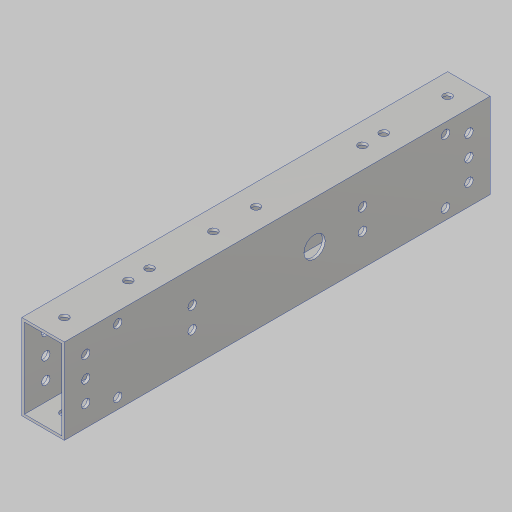
# Autodesk Inventor part: EL2-C-005
Saved by Autodesk Inventor 2023.5 (Build 275446000, 446)
## iProperties
RuleStatus: InUse
Created: 2025-01-11
Part Number: EL2-C-005
Material: Aluminum 6061
Document SubType Name: Modeling
Designer: brand
Mass: 304.185 g
Surface Area: 718.547 cm^2
Volume: 112.661 cm^3
Density: 2.7 g/cm^3
Appearance: Aluminum - Flat
AfterDocNew0: SHOW
AfterDocOpen0: SHOW
Author: brand
Autodesk Inventor part; units mm, degrees
ref_plane "YZ Plane" through (0, 0, 0) normal (1, 0, 0) x (0, 1, 0)
ref_plane "XZ Plane" through (0, 0, 0) normal (0, 1, 0) x (-1, 0, 0)
ref_plane "XY Plane" through (0, 0, 0) normal (0, 0, 1) x (1, 0, 0)
sketch "Sketch1" plane through (0, 0, 0) normal (0, 0, 1) x (1, 0, 0)
  line L0 (-12.7, -25.4) -> (12.7, -25.4)
  line L1 (12.7, -25.4) -> (12.7, 25.4)
  line L2 (12.7, 25.4) -> (-12.7, 25.4)
  line L3 (-12.7, 25.4) -> (-12.7, -25.4)
  line L4 (-12.7, -25.4) -> (12.7, 25.4) construction
  line L5 (12.7, -25.4) -> (-12.7, 25.4) construction
  line L6 (-11.1125, 23.8125) -> (11.1125, 23.8125)
  line L7 (11.1125, 23.8125) -> (11.1125, -23.8125)
  line L8 (11.1125, -23.8125) -> (-11.1125, -23.8125)
  line L9 (-11.1125, -23.8125) -> (-11.1125, 23.8125)
  point P0 (0, 0)
  dimension "width" = 25.4
  dimension "height" = 50.8
  dimension "thickness" = 1.5875
  constraints: 20 end point, 4 parallel, 2 midpoint, 2 perpendicular, 1 horizontal, 3 other
  measures "width" distance of L2.end L1.end
  measures "height" distance of L1.end L0.end
  measures "thickness" distance between parallel lines of L2 L6
extrude "Extrusion1" add sketch "Sketch1" along normal mid plane 254
sketch "Sketch2" plane through (-12.7, -25.4, 127) normal (-1, 0, 0) x (0, 0, 1)
  line L0 (-254, 0) -> (-254, 50.8) construction
  line L1 (-254, 50.8) -> (0, 50.8) construction
  line L2 (0, 50.8) -> (0, 0) construction
  line L3 (0, 0) -> (-254, 0) construction
  point P0 (-127, 25.4)
  point P1 (-241.3, 38.1)
  point P2 (-241.3, 25.4)
  point P3 (-241.3, 12.7)
  point P4 (-12.7, 38.1)
  point P5 (-12.7, 25.4)
  point P6 (-12.7, 12.7)
  point P7 (-254, 25.4)
  dimension "d5" = 12.7
  dimension "d6" = 12.7
  dimension "d7" = 12.7
  dimension "d8" = 12.7
  constraints: 4 horizontal alignment, 4 vertical alignment, 1 midpoint
  measures "d5" distance of point (-241.3, 38.1) point (-241.3, 25.4)
  measures "d6" distance of point (-241.3, 12.7) point (-241.3, 25.4)
  measures "d7" distance from line of L0 point (-241.3, 25.4)
  measures "d8" distance from line of L2 point (-12.7, 25.4)
hole "Block Mount Holes" at (-12.7, 12.7, -114.3) at (-12.7, 0, -114.3) at (-12.7, -12.7, -114.3) at (-12.7, 12.7, 114.3) at (-12.7, 0, 114.3) at (-12.7, -12.7, 114.3) direction (1, 0, 0) diameter 5.1054 end through all clearance for "Flat Head Machine Screw (82)" size "#10" standard "Ansi Unified Screw Threads"
sketch "Sketch4" plane through (-12.7, 25.4, 127) normal (0, 1, 0) x (1, 0, 0)
  line L0 (0, 254) -> (25.4, 254) projected
  line L1 (12.7, 190.5) -> (12.7, 63.5) construction
  point P0 (12.7, 127)
  point P1 (12.7, 254)
  point P2 (12.7, 203.2)
  point P3 (12.7, 50.8)
  point P4 (12.7, 127)
  dimension "d61" = 12.7
  dimension "d65" = 127
  dimension "d66" = 12.7
  constraints: 3 vertical alignment, 2 end point, 2 midpoint, 1 coincident, 1 vertical
  measures "d61" distance of point (12.7, 203.2) L1.start
  measures "d65" distance of L1.end L1.start
  measures "d66" distance of L1.end point (12.7, 50.8)
hole "Hole3" at (0, 25.4, 63.5) at (0, 25.4, -63.5) at (0, 25.4, -76.2) at (0, 25.4, 76.2) direction (0, -1, 0) diameter 5.1054 end through all clearance for "Flat Head Machine Screw (82)" size "#10" standard "Ansi Unified Screw Threads"
sketch "Sketch8" plane through (-12.7, 25.4, 127) normal (0, 1, 0) x (1, 0, 0)
  circle A0 centre (12.7, 203.2) radius 2.5527 construction
  circle A1 centre (12.7, 63.5) radius 2.5527 construction
  circle A2 centre (12.7, 190.5) radius 2.5527 construction
  circle A3 centre (12.7, 50.8) radius 2.5527 construction
  line L0 (0, 254) -> (25.4, 254) construction
  line L1 (25.4, 254) -> (25.4, 0) construction
  line L2 (25.4, 0) -> (0, 0) construction
  line L3 (0, 0) -> (0, 254) construction
  point P0 (12.7, 127)
  point P1 (12.7, 127)
  point P2 (12.7, 101.6)
  point P3 (9.9314, 152.4)
  dimension "d67" = 25.4
  dimension "d68" = 25.4
  constraints: 1 coincident, 1 vertical alignment
  measures "d67" distance of point (12.7, 101.6) point (12.7, 127)
  measures "d68" vertical distance of point (9.931, 152.4) point (12.7, 127)
hole "Hole5" at (0, 25.4, 0) at (0, 25.4, 25.4) direction (0, -1, 0) diameter 5.1054 end through all clearance for "Flat Head Machine Screw (82)" size "#10" standard "Ansi Unified Screw Threads"
sketch "Sketch9" plane through (-12.7, 25.4, 127) normal (0, 1, 0) x (1, 0, 0)
  line L0 (0, 254) -> (25.4, 254) projected
  line L1 (25.4, 0) -> (0, 0) projected
  point P0 (12.7, 127)
  point P1 (12.7, 12.7)
  point P2 (12.7, 241.3)
  point P3 (12.7, 254)
  point P4 (12.7, 254)
  point P5 (12.7, 0)
  dimension "d79" = 12.7
  dimension "d80" = 12.7
  constraints: 3 midpoint, 2 vertical alignment
  measures "d79" distance of point (12.7, 254) point (12.7, 241.3)
  measures "d80" distance from line of L1 point (12.7, 12.7)
hole "Hole6" at (0, 25.4, 114.3) at (0, 25.4, -114.3) direction (0, -1, 0) diameter 5.1054 end through all clearance for "Flat Head Machine Screw (82)" size "#10" standard "Ansi Unified Screw Threads"
sketch "Sketch10" plane through (12.7, -25.4, 127) normal (1, 0, 0) x (0, 0, -1)
  line L0 (254, 50.8) -> (254, 0) projected
  line L1 (184.15, 40.3225) -> (184.15, 10.4775) construction
  point P0 (127, 25.4)
  point P1 (184.15, 25.4)
  point P2 (254, 25.4)
  point P3 (149.225, 25.4)
  point P4 (254, 25.4)
  dimension "d88" = 69.85
  dimension "d89" = 29.845
  dimension "d97" = 104.775
  constraints: 3 midpoint, 2 end point, 2 horizontal alignment, 1 vertical, 1 vertical alignment
  measures "d88" distance from line of L0 L1.start
  measures "d89" distance of L1.start L1.end
  measures "d97" distance of point (254, 25.4) point (149.225, 25.4)
hole "Hole8" at (12.7, 0, -22.225) direction (-1, 0, 0) diameter 5.1054 end through all clearance for "Flat Head Machine Screw (82)" size "#10" standard "Ansi Unified Screw Threads"
sketch "Sketch11" plane through (12.7, -25.4, 127) normal (1, 0, 0) x (0, 0, -1)
  line L0 (76.2, 31.75) -> (76.2, 19.05) construction
  line L1 (0, 0) -> (0, 50.8) construction
  point P0 (127, 25.4)
  point P1 (76.2, 25.4)
  point P2 (0, 25.4)
  dimension "d105" = 76.2
  dimension "d106" = 12.7
  constraints: 2 end point, 2 midpoint, 1 horizontal alignment, 1 vertical, 1 vertical alignment
  measures "d105" distance from line of L1 L0.start
  measures "d106" distance of L0.start L0.end
hole "Hole9" at (12.7, 6.35, 50.8) at (12.7, -6.35, 50.8) direction (-1, 0, 0) diameter 5.1054 end through all clearance for "Flat Head Machine Screw (82)" size "#10" standard "Ansi Unified Screw Threads"
mirror "Mirror1" about plane through (0, 0, 0) normal (0, 0, 1) of "Hole9"
sketch "Sketch13" plane through (12.7, -25.4, 127) normal (1, 0, 0) x (0, 0, -1)
  circle A0 centre (177.8, 19.05) radius 2.5527 projected
  circle A1 centre (177.8, 31.75) radius 2.5527 projected
  circle A2 centre (76.2, 31.75) radius 2.5527 projected
  circle A3 centre (76.2, 19.05) radius 2.5527 projected
  circle A4 centre (149.225, 25.4) radius 2.5527 projected
  circle A5 centre (12.7, 25.4) radius 2.5527 projected
  circle A6 centre (241.3, 12.7) radius 2.5527 projected
  circle A7 centre (241.3, 38.1) radius 2.5527 projected
  circle A8 centre (241.3, 25.4) radius 2.5527 projected
  circle A9 centre (12.7, 38.1) radius 2.5527 projected
  circle A10 centre (12.7, 12.7) radius 2.5527 projected
  line L0 (254, 50.8) -> (254, 0) projected
  line L1 (254, 0) -> (0, 0) projected
  line L2 (0, 0) -> (0, 50.8) projected
  line L3 (0, 50.8) -> (254, 50.8) projected
  circle A11 centre (149.225, 25.4) radius 2.5527 projected
  circle A12 centre (149.225, 25.4) radius 6.35
  point P0 (127, 25.4)
  dimension "d117" = 12.7
  constraints: 1 centre point, 1 coincident
  measures "d117" diameter of A12
extrude "Extrusion5" cut sketch "Sketch13" against normal up to surface (1.5875 mm away) contours A12
sketch "Sketch14" plane through (12.7, -25.4, 127) normal (1, 0, 0) x (0, 0, -1)
  line L0 (227.3376, 44.45) -> (227.3376, 6.35) construction
  line L1 (254, 50.8) -> (254, 0) construction
  line L2 (31.75, 44.45) -> (31.75, 6.35) construction
  line L3 (0, 0) -> (0, 50.8) construction
  point P0 (127, 25.4)
  point P1 (227.3376, 25.4)
  point P2 (254, 25.4)
  point P3 (31.75, 25.4)
  point P4 (0, 25.4)
  dimension "d120" = 38.1
  dimension "d121" = 26.6624
  dimension "d129" = 38.1
  dimension "d130" = 31.75
  constraints: 4 end point, 4 midpoint, 2 horizontal alignment, 2 vertical, 1 coincident, 1 vertical alignment
  measures "d120" distance of L0.start L0.end
  measures "d121" distance between parallel lines of L1 L0
  measures "d129" distance of L2.start L2.end
  measures "d130" distance between parallel lines of L3 L2
hole "Hole10" at (12.7, 19.05, -100.3376) at (12.7, -19.05, -100.3376) at (12.7, 19.05, 95.25) at (12.7, -19.05, 95.25) direction (-1, 0, 0) diameter 5.1054 end through all clearance for "Flat Head Machine Screw (82)" size "#10" standard "Ansi Unified Screw Threads"
equation "\"d6\" = d5"
equation "\"d8\" = d7"
equation "\"d80\" = d79"
body "Solid1"
